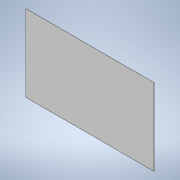
# Autodesk Inventor part: Aluminium_Grundplatte
Saved by Autodesk Inventor 2020 (Build 240168000, 168)
## iProperties
Created: 2023-11-19
Part Number: Aluminium_Grundplatte
Material: Aluminum 6061-AHC
Document SubType Name: Modeling
Designer: haniv
Density: 2.7 g/cm^3
Appearance: Aluminium - dunkel
Author: haniv
Autodesk Inventor part; units mm, degrees
ref_plane "YZ Plane" through (0, 0, 0) normal (1, 0, 0) x (0, 1, 0)
ref_plane "XZ Plane" through (0, 0, 0) normal (0, 1, 0) x (-1, 0, 0)
ref_plane "XY Plane" through (0, 0, 0) normal (0, 0, 1) x (1, 0, 0)
sketch "Skizze1" plane through (0, 0, 0) normal (0, 0, 1) x (1, 0, 0)
  line L0 (-500, 300) -> (500, 300)
  line L1 (500, 300) -> (500, -300)
  line L2 (500, -300) -> (-500, -300)
  line L3 (-500, -300) -> (-500, 300)
  point P0 (0, 0)
  point P1 (0, 300)
  point P2 (-500, 0)
  dimension "d0" = 1000
  dimension "d1" = 600
  constraints: 8 end point, 2 midpoint, 2 parallel, 1 horizontal, 1 horizontal alignment, 1 perpendicular, 1 vertical alignment
  measures "d0" distance of L1.end L2.end
  measures "d1" distance of L0.end L1.end
extrude "Extrusion1" add sketch "Skizze1" along normal blind 1
